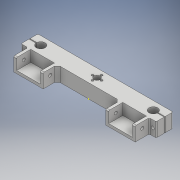
# Autodesk Inventor part: Trava Z
Saved by Autodesk Inventor 2017 (Build 210142000, 142)
## iProperties
Created: 2020-08-03
Part Number: Trava Z
Material: Generic
Document SubType Name: Modeling
Designer: ale
Density: 1 g/cm^3
Appearance: Default
Author: ale
Autodesk Inventor part; units mm, degrees
ref_plane "YZ Plane" through (0, 0, 0) normal (1, 0, 0) x (0, 1, 0)
ref_plane "XZ Plane" through (0, 0, 0) normal (0, 1, 0) x (-1, 0, 0)
ref_plane "XY Plane" through (0, 0, 0) normal (0, 0, 1) x (1, 0, 0)
sketch "Sketch1" plane through (0, 0, 0) normal (0, 0, 1) x (1, 0, 0)
  line L0 (-120, 15) -> (120, 15)
  line L1 (120, -15) -> (-120, -15)
  line L2 (-120, 15) -> (120, -15) construction
  line L3 (120, 15) -> (-120, -15) construction
  arc A0 (-107.7136, -0.75) -> (-107.7136, 0.75) centre (-100, 0) ccw
  line L4 (0, -11.513) -> (0, 11.513)
  line L5 (-107.7136, 0.75) -> (-120, 0.75)
  line L6 (-107.7136, -0.75) -> (-120, -0.75)
  line L7 (-120, -15) -> (-120, -0.75)
  line L8 (-120, 0.75) -> (-120, 15)
  arc A1 (107.7136, 0.75) -> (107.7136, -0.75) centre (100, 0) ccw
  line L9 (107.7136, 0.75) -> (120, 0.75)
  line L10 (107.7136, -0.75) -> (120, -0.75)
  line L11 (120, 15) -> (120, 0.75)
  line L12 (120, -0.75) -> (120, -15)
  circle A2 centre (0, 0) radius 5.5
  circle A3 centre (0, 8) radius 2
  circle A4 centre (8, 0) radius 2
  circle A5 centre (0, -8) radius 2
  circle A6 centre (-8, 0) radius 2
  dimension "d0" = 240
  dimension "d1" = 30
  dimension "d3" = 15.5
  dimension "d6" = 100
  dimension "d7" = 11
  dimension "d9" = 4
  dimension "d10" = 4
  dimension "d11" = 4
  dimension "d12" = 4
  constraints: 26 end point, 7 centre point, 5 parallel, 5 symmetric about line, 4 midpoint, 4 point on circle, 2 perpendicular, 2 point on line, 1 coincident, 1 horizontal, 1 vertical, 1 other
  measures "d0" distance of L1.start L1.end
  measures "d1" distance of L0.end L1.start
  measures "d3" diameter of A0
  measures "d6" distance of A0.centre point (0, 0)
  measures "d7" diameter of A2
  measures "d9" diameter of A3
  measures "d10" diameter of A4
  measures "d11" diameter of A5
  measures "d12" diameter of A6
extrude "Extrusion1" add sketch "Sketch1" along normal blind 25
sketch "Sketch2" plane through (-120, -15, 0) normal (0, -1, 0) x (1, 0, 0)
  line L0 (120, 0) -> (120, 25)
  line L1 (12.2864, 0) -> (12.2864, 25) projected
  line L2 (0, 25) -> (240, 25) projected
  line L3 (12.2864, 0) -> (64.2864, 0)
  line L4 (64.2864, 0) -> (64.2864, 25)
  line L5 (12.2864, 25) -> (12.2864, 0)
  line L6 (59.2864, 25) -> (59.2864, 5)
  line L7 (59.2864, 5) -> (17.2864, 5)
  line L8 (17.2864, 5) -> (17.2864, 25)
  line L9 (64.2864, 25) -> (59.2864, 25)
  line L10 (17.2864, 25) -> (12.2864, 25)
  line L11 (227.7136, 0) -> (227.7136, 25)
  line L12 (240, 25) -> (0, 25)
  line L13 (227.7136, 0) -> (175.7136, 0)
  line L14 (175.7136, 0) -> (175.7136, 25)
  line L15 (227.7136, 25) -> (227.7136, 0)
  line L16 (180.7136, 25) -> (180.7136, 5)
  line L17 (180.7136, 5) -> (222.7136, 5)
  line L18 (222.7136, 5) -> (222.7136, 25)
  line L19 (175.7136, 25) -> (180.7136, 25)
  line L20 (222.7136, 25) -> (227.7136, 25)
  line L21 (240, 0) -> (0, 0) projected
  dimension "d23" = 52
  dimension "d24" = 5
  dimension "d28" = 0
  dimension "d30" = 20
  constraints: 38 end point, 12 symmetric about line, 4 parallel, 2 perpendicular, 2 point on line, 1 horizontal, 1 vertical
  measures "d23" distance of L5.start L4.end
  measures "d24" distance between parallel lines of L4 L6
  measures "d28" vertical distance of L2.start L5.start
  measures "d30" distance between parallel lines of L2 L7
sketch "Sketch3" plane through (120, -15, 0) normal (0, -1, 0) x (1, 0, 0)
  point P0 (-120, 0)
extrude "Extrusion4" add sketch "Sketch2" along normal blind 25 contours L14 L2 L16 L17 L18 L11 L13 | L3 L1 L2 L8 L7 L6 L4
sketch "Sketch4" plane through (120, -15, 0) normal (0, -1, 0) x (1, 0, 0)
  line L0 (-240, 0) -> (0, 0) projected
  line L1 (-12.2864, 25) -> (0, 25) projected
  circle A0 centre (-6.1432, 12.5) radius 2.75
  line L2 (-120, 0) -> (-120, 25)
  line L3 (-122, 0) -> (-122, 25) projected
  circle A1 centre (-233.8568, 12.5) radius 2.75
  dimension "d33" = 5.5
  constraints: 2 centre point, 2 end point, 1 parallel, 1 symmetric about line, 1 other
  measures "d33" diameter of A0
hole "Hole1" at (113.8568, -15, 12.5) at (-113.8568, -15, 12.5) direction (0, 1, 0) diameter 5.5 end through all
sketch "Sketch5" plane through (-107.7136, -15, 0) normal (-1, 0, 0) x (0, 0, 1)
  line L0 (5, 0) -> (5, -25) projected
  line L1 (5, 0) -> (24.9936, -25)
  circle A0 centre (14.9968, -12.5) radius 2.75
  point P0 (0, 15)
  dimension "d41" = 5.5
  constraints: 2 end point, 1 centre point, 1 midpoint
  measures "d41" diameter of A0
extrude "Extrusion5" cut sketch "Sketch5" against normal through all
chamfer "Chamfer2" distance 5 angle 45 2 edges at (-55.7136, -15, 12.5) (55.7136, -15, 12.5)
chamfer "Chamfer3" distance 2 angle 45 2 edges at (-107.7136, -15, 12.5) (107.7136, -15, 12.5)
fillet "Fillet2" radius 2 8 edges at (120, -15, 12.5) (120, 15, 12.5) (105.2136, -40, 25) (58.2136, -40, 25) (-58.2136, -40, 25) (-105.2136, -40, 25) (-120, -15, 12.5) (-120, 15, 12.5)
body "Solid1"
